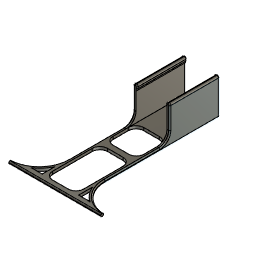
pipette uprighter wide 28mm (Autodesk Fusion 360 design; units mm, degrees)
Autodesk Fusion 360 part; units mm, degrees
sketch "Sketch1" plane through (0, 0, 0) normal (0, 0, 1) x (1, 0, 0)
  line L0 (16.5, -22.5) -> (-16.5, -22.5)
  line L1 (-16.5, -22.5) -> (-16.5, 22.5)
  line L2 (-16.5, 22.5) -> (16.5, 22.5)
  line L3 (16.5, 22.5) -> (16.5, -22.5)
  line L4 (16.5, -22.5) -> (-16.5, 22.5) construction
  line L5 (-16.5, -22.5) -> (16.5, 22.5) construction
  line L6 (14, 22.5) -> (-14, 22.5)
  line L7 (-14, 22.5) -> (-14, -22.5)
  line L8 (-14, -22.5) -> (14, -22.5)
  line L9 (14, -22.5) -> (14, 22.5)
  line L10 (14, 22.5) -> (-14, -22.5) construction
  line L11 (-14, 22.5) -> (14, -22.5) construction
  line L12 (-16.5, -22.5) -> (-14, -22.5)
  line L13 (-14, -22.5) -> (-14, -107.5)
  line L14 (-14, -107.5) -> (-16.5, -107.5)
  line L15 (-16.5, -107.5) -> (-16.5, -22.5)
  line L16 (14, -22.5) -> (16.5, -22.5)
  line L17 (16.5, -22.5) -> (16.5, -107.5)
  line L18 (16.5, -107.5) -> (14, -107.5)
  line L19 (14, -107.5) -> (14, -22.5)
  line L20 (-14, -50.1945) -> (14, -50.1945)
  line L21 (14, -50.1945) -> (14, -55.1945)
  line L22 (14, -55.1945) -> (-14, -55.1945)
  line L23 (-14, -55.1945) -> (-14, -50.1945)
  arc A0 (-41.5, -107.4946) -> (-16.5, -81.136) centre (-42.8956, -81.136) ccw
  arc A1 (16.5, -81.105) -> (41.4999, -107.4229) centre (42.8526, -81.105) ccw
  arc A2 (16.5, -92.2652) -> (31.4998, -107.4315) centre (42.0559, -81.9906) ccw
  arc A3 (-31.5, -107.486) -> (-16.5, -93.4519) centre (-41.6221, -81.634) ccw
  line L24 (-41.5, -107.4946) -> (41.4999, -107.4229)
  line L25 (41.4999, -109.9229) -> (-41.5, -109.9946)
  line L26 (-41.5, -109.9946) -> (-41.5, -107.4946)
  line L27 (41.4999, -109.9229) -> (41.4999, -107.4229)
  dimension "d1" = 33
  dimension "d2" = 45
  dimension "d3" = 28
  dimension "d4" = 45
  dimension "d5" = 2.5
  dimension "d6" = 85
  dimension "d7" = 2.5
  dimension "d8" = 5
  dimension "d9" = 25
  dimension "d10" = 25
  dimension "d11" = 15
  dimension "d12" = 15
  dimension "d13" = 2.5
  constraint horizontal L0
  constraint perpendicular L0 L1
  constraint parallel L0 L2
  constraint parallel L1 L3
  constraint coincident L4 origin
  constraint coincident L5 origin
  constraint horizontal L6
  constraint perpendicular L6 L7
  constraint parallel L6 L8
  constraint parallel L7 L9
  constraint coincident L10 origin
  constraint coincident L11 origin
  constraint horizontal L12
  constraint vertical L13
  constraint horizontal L14
  constraint vertical L15
  constraint horizontal L16
  constraint vertical L17
  constraint horizontal L18
  constraint vertical L19
  constraint horizontal L20
  constraint vertical L21
  constraint horizontal L22
  constraint vertical L23
  constraint coincident L13 L20.start
  constraint tangent L15 A0
  constraint coincident L15 A0.end
  constraint tangent L17 A1
  constraint coincident L17 A1.start
  constraint tangent A1 A2
  constraint coincident L17 A2.start
  constraint tangent A0 A3
  constraint coincident L15 A3.end
  constraint parallel L24 L25
  constraint vertical L26
  constraint parallel L26 L27
  constraint coincident A2.end L24
  constraint coincident A3.start L24
  measures "d1" distance of L1.end L2.end
  measures "d2" distance of L0.end L1.end
  measures "d3" distance of L7.end L8.end
  measures "d4" distance of L6.end L7.end
  measures "d5" distance of L0.end L7.end
  measures "d6" distance of L0.end L14.end
  measures "d7" distance of L8.end L0.start
  measures "d8" distance of L20.start L22.end
  measures "d9" distance of L14.end A0.start
  measures "d10" distance of L17.end A1.end
  measures "d11" distance of L14.end A3.start
  measures "d12" distance of L17.end A2.end
  measures "d13" distance of A1.end L25.start
extrude "Extrude1" add sketch "Sketch1" along normal blind 30 contours L0 L2 L3 L9 L16 | L0 L1 L2 L7 L12 makes body 1 at (-16.5, -7.5, 10) makes body 2 at (14, -7.5, 10)
extrude "Extrude2" add sketch "Sketch1" against normal blind 2.5 separate body contours L0 L16 L17 L19 L21 L24 | L0 L2 L3 L9 L16 | L0 L2 L6 L7 L8 L9 | L0 L12 L13 L15 L23 L24 | L0 L1 L2 L7 L12 | L13 L19 L20 L21 L22 L23 | L13 L14 L15 L17 L18 L19 L24 L25 L26 L27 makes body 3 at (-4.6667, 7.5, 0)
extrude "Extrude3" add sketch "Sketch1" against normal blind 2.5 separate body contours L15 A0 A3 L24 makes body 4
extrude "Extrude4" add sketch "Sketch1" against normal blind 2.5 separate body contours L17 A1 A2 L24 makes body 5
sketch "Sketch2" plane through (0, -22.5, 0) normal (0, -1, 0) x (1, 0, 0)
  line L0 (-16.5, 0) -> (-14, 0)
  line L1 (-14, 0) -> (-14, 30)
  line L2 (-14, 30) -> (-16.5, 30)
  line L3 (-16.5, 30) -> (-16.5, 0)
  line L4 (-14, 30) -> (-13, 30)
  line L5 (-13, 30) -> (-13, 25)
  line L6 (-13, 25) -> (-14, 25)
  line L7 (-14, 25) -> (-14, 30)
  constraint horizontal L4
  constraint vertical L5
  constraint horizontal L6
  constraint vertical L7
  constraint coincident L1.end L2.start
sketch "Sketch5" plane through (0, -22.5, 0) normal (0, -1, 0) x (1, 0, 0)
  line L0 (14, 0) -> (16.5, 0)
  line L1 (16.5, 0) -> (16.5, 30)
  line L2 (16.5, 30) -> (14, 30)
  line L3 (14, 30) -> (14, 0)
  line L4 (14, 30) -> (13, 30)
  line L5 (13, 30) -> (13, 25)
  line L6 (13, 25) -> (14, 25)
  line L7 (14, 25) -> (14, 30)
  constraint horizontal L4
  constraint vertical L5
  constraint horizontal L6
  constraint vertical L7
  constraint coincident L2.end L3.start
extrude "Extrude6" add sketch "Sketch5" sketch "Sketch2" along normal up to surface contours L3 L4 L5 L6 L7 of sketch 2 contours L1 L4 L5 L6 L7 end surface through (14, 22.5, 0) normal (0, 1, 0) offset 0 bodies 1 2 3 4 5
fillet "Fillet1" radius 2.5 2 edges at (-13, 0, 25) (13, 0, 25) on bodies 1 2
fillet "Fillet1" radius 1.5 4 edges at (-13, 0, 30) (-16.5, 0, 30) (13, 0, 30) (16.5, 0, 30) on bodies 1 2
fillet "Fillet2" radius 1 2 edges at (16.5, 22.5, -1.25) (-16.5, 22.5, -1.25) on bodies 3
combine "Combine1" operation add target body 1 tool bodies 4 5 3 2
sketch "Sketch6" plane through (16.5, 0, 0) normal (1, 0, 0) x (0, 1, 0)
  line L0 (-81.105, 0) -> (-81.105, -2.5)
  line L1 (-81.105, -2.5) -> (21.5, -2.5)
  line L2 (21.5, -2.5) -> (21.5, 0)
  line L3 (21.5, 0) -> (22.5, 0)
  line L4 (22.5, 0) -> (22.5, 28.5)
  line L5 (22.5, 28.5) -> (-22.5, 28.5)
  line L6 (-22.5, 28.5) -> (-22.5, 0)
  line L7 (-22.5, 0) -> (-81.105, 0)
fillet "Fillet3" radius 9 2 edges at (15.25, -22.5, 0) (-15.25, -22.5, 0) on bodies 1
fillet "Fillet3" radius 7 4 edges at (-14, -22.5, -1.25) (14, -22.5, -1.25) (-14, -50.1945, -1.25) (14, -50.1945, -1.25) on bodies 1
fillet "Fillet3" radius 7 4 edges at (14, -55.1945, -1.25) (-14, -55.1945, -1.25) (-14, -107.4708, -1.25) (14, -107.4467, -1.25) on bodies 1
sketch "Sketch7" plane through (0, 0, -2.5) normal (0, 0, -1) x (1, 0, 0)
  arc A0 (-16.5, 93.4519) -> (-31.5, 107.486) centre (-41.6221, 81.634) ccw
  line L0 (-31.5, 107.486) -> (-16.5, 107.473)
  line L1 (-16.5, 107.473) -> (-16.5, 107.5)
  line L2 (-16.5, 107.5) -> (-14, 107.5)
  line L3 (-14, 107.5) -> (-14, 107.4708)
  line L4 (-14, 107.4708) -> (14, 107.4467)
  line L5 (14, 107.4467) -> (14, 107.5)
  line L6 (14, 107.5) -> (16.5, 107.5)
  line L7 (16.5, 107.5) -> (16.5, 107.4445)
  line L8 (16.5, 107.4445) -> (31.4998, 107.4315)
  arc A1 (31.4998, 107.4315) -> (16.5, 92.2652) centre (42.0559, 81.9906) ccw
  line L9 (16.5, 92.2652) -> (16.5, 107.4445)
  line L10 (16.5, 107.4445) -> (14, 107.4467)
  line L11 (14, 107.4467) -> (14, 62.1945)
  arc A2 (7, 55.1945) -> (14, 62.1945) centre (7, 62.1945) ccw
  line L12 (7, 55.1945) -> (-7, 55.1945)
  arc A3 (-14, 62.1945) -> (-7, 55.1945) centre (-7, 62.1945) ccw
  line L13 (-14, 62.1945) -> (-14, 107.4708)
  line L14 (-14, 107.4708) -> (-16.5, 107.473)
  line L15 (-16.5, 107.473) -> (-16.5, 93.4519)
  line L16 (-14, 29.5) -> (-14, 43.1945)
  arc A4 (-7, 50.1945) -> (-14, 43.1945) centre (-7, 43.1945) ccw
  line L17 (-7, 50.1945) -> (7, 50.1945)
  arc A5 (14, 43.1945) -> (7, 50.1945) centre (7, 43.1945) ccw
  line L18 (14, 43.1945) -> (14, 29.5)
  arc A6 (7, 22.5) -> (14, 29.5) centre (7, 29.5) ccw
  line L19 (7, 22.5) -> (-7, 22.5)
  arc A7 (-14, 29.5) -> (-7, 22.5) centre (-7, 29.5) ccw
  line L20 (-16.5, 81.136) -> (-16.5, -21.5)
  arc A8 (-16.5, -21.5) -> (-15.5, -22.5) centre (-15.5, -21.5) ccw
  line L21 (-15.5, -22.5) -> (15.5, -22.5)
  arc A9 (15.5, -22.5) -> (16.5, -21.5) centre (15.5, -21.5) ccw
  line L22 (16.5, -21.5) -> (16.5, 81.105)
  arc A10 (41.4999, 107.4229) -> (16.5, 81.105) centre (42.8526, 81.105) ccw
  line L23 (41.4999, 107.4229) -> (41.4999, 109.9229)
  line L24 (41.4999, 109.9229) -> (-41.5, 109.9946)
  line L25 (-41.5, 109.9946) -> (-41.5, 107.4946)
  arc A11 (-16.5, 81.136) -> (-41.5, 107.4946) centre (-42.8956, 81.136) ccw
  line L26 (-31.5, 109.986) -> (31.4998, 109.986)
  line L27 (31.4998, 109.986) -> (31.4998, 104.8868)
  line L28 (31.4998, 104.8868) -> (-31.5, 104.8868)
  line L29 (-31.5, 104.8868) -> (-31.5, 109.986)
  constraint horizontal L26
  constraint vertical L27
  constraint horizontal L28
  constraint vertical L29
  constraint coincident A10 L27.end
  constraint coincident L24 L26.start
extrude "Extrude7" add sketch "Sketch7" against normal blind 2.5 contours A0 L0 L15 L28 | L13 L14 L15 L28 | L0 L1 L2 L3 L4 L5 L6 L7 L8 L24 L27 L29 | L1 L2 L3 L14 | L4 L11 L13 L28 | L9 L10 L11 L28 | L5 L6 L7 L10 | L8 A1 L9 L28 bodies 1
fillet "Fillet4" radius 7 2 edges at (14, -104.8868, -1.25) (-14, -104.8868, -1.25) on bodies 1
fillet "Fillet5" radius 1 7 edges at (-23.744, -99.3003, -2.5) (-16.5, -29.818, -2.5) (-16.2071, 22.2071, -2.5) (0, 22.5, -2.5) (16.2071, 22.2071, -2.5) (16.5, -29.8025, -2.5) (23.7462, -99.2546, -2.5) on bodies 1
fillet "Fillet5" radius 1 15 edges at (-16.5, 22.5, 14.25) (-16.0607, 22.5, 29.5607) (-14.75, 22.5, 30) (-13.4393, 22.5, 29.5607) (-13, 22.5, 27.75) (-13.2639, 22.5, 25.882) (16.5, 22.5, 14.25) (16.0607, 22.5, 29.5607) (14.75, 22.5, 30) (13.4393, 22.5, 29.5607) (13, 22.5, 27.75) (13.2639, 22.5, 25.882) (14, 22.5, 12.5) (-14, 22.5, 12.5) (0, 22.5, 0) on bodies 1
fillet "Fillet5" radius 1 18 edges at (-23.744, -99.3003, 0) (-16.5, -56.318, 0) (-16.5, -25.136, 2.636) (-16.5, -22.5, 18.75) (-16.0607, -22.5, 29.5607) (-14.75, -22.5, 30) (-13.4393, -22.5, 29.5607) (-13, -22.5, 27.75) (-13.2639, -22.5, 25.882) (23.7462, -99.2546, 0) (16.5, -56.3025, 0) (16.5, -25.136, 2.636) (16.5, -22.5, 18.75) (16.0607, -22.5, 29.5607) (14.75, -22.5, 30) (13.4393, -22.5, 29.5607) (13, -22.5, 27.75) (13.2639, -22.5, 25.882) on bodies 1
fillet "Fillet5" radius 1 2 edges at (-0.0001, -109.9587, -2.5) (-0.0001, -109.9587, 0) on bodies 1
equation "d3 = 33 mm - 5 mm"
